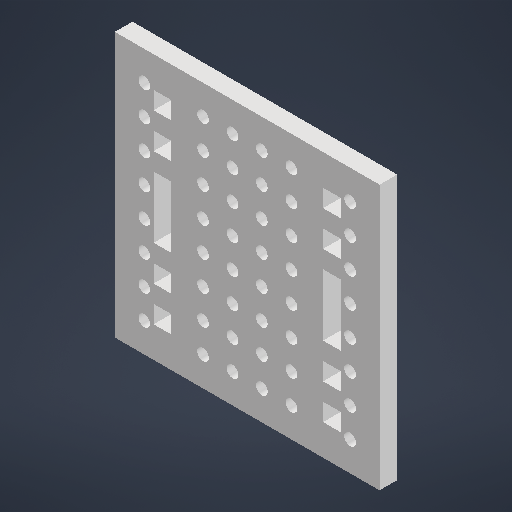
# Autodesk Inventor part: FootScrewplate
Saved by Autodesk Inventor 2027 (Build 310192000, 192)
## iProperties
Created: 2026-04-15
Part Number: FootScrewplate
Material: Generic
Document SubType Name: Modeling
Designer: Tueha
Density: 1 g/cm^3
Appearance: Default
Author: Tueha
Autodesk Inventor part; units mm, degrees
ref_plane "YZ Plane" through (0, 0, 0) normal (1, 0, 0) x (0, 1, 0)
ref_plane "XZ Plane" through (0, 0, 0) normal (0, 1, 0) x (-1, 0, 0)
ref_plane "XY Plane" through (0, 0, 0) normal (0, 0, 1) x (1, 0, 0)
sketch "Sketch1" plane through (0, 0, 0) normal (0, 0, 1) x (1, 0, 0)
  line L0 (-43.8671, 76.4402) -> (46.1329, 76.4402)
  line L1 (46.1329, 76.4402) -> (46.1329, -13.5598)
  line L2 (46.1329, -13.5598) -> (-43.8671, -13.5598)
  line L3 (-43.8671, -13.5598) -> (-43.8671, 76.4402)
  point P0 (0, 0)
  dimension "d0" = 90
  dimension "d1" = 90
  constraints: 8 end point, 2 parallel, 1 horizontal, 1 perpendicular
  measures "d0" distance of L1.end L2.end
  measures "d1" distance of L0.end L1.end
extrude "Extrusion1" add sketch "Sketch1" along normal blind 6
sketch "Sketch2" plane through (0, 0, 0) normal (0, 0, -1) x (-1, 0, 0)
  line L0 (24.6671, 8.9402) -> (30.6671, 8.9402) projected
  line L1 (30.6671, 8.9402) -> (30.6671, 2.9402) projected
  line L2 (30.6671, 2.9402) -> (24.6671, 2.9402) projected
  line L3 (24.6671, 8.9402) -> (24.6671, 2.9402) projected
  line L4 (30.6671, 14.9402) -> (24.6671, 14.9402) projected
  line L5 (24.6671, 20.9402) -> (24.6671, 14.9402) projected
  line L6 (30.6671, 20.9402) -> (24.6671, 20.9402) projected
  line L7 (30.6671, 20.9402) -> (30.6671, 14.9402) projected
  line L8 (24.6671, 47.9402) -> (30.6671, 47.9402) projected
  line L9 (30.6671, 41.9402) -> (30.6671, 47.9402) projected
  line L10 (24.6671, 41.9402) -> (30.6671, 41.9402) projected
  line L11 (24.6671, 41.9402) -> (24.6671, 47.9402) projected
  line L12 (24.6671, 59.9402) -> (30.6671, 59.9402) projected
  line L13 (30.6671, 53.9402) -> (30.6671, 59.9402) projected
  line L14 (30.6671, 53.9402) -> (24.6671, 53.9402) projected
  line L15 (24.6671, 53.9402) -> (24.6671, 59.9402) projected
  line L16 (-32.9329, 47.9402) -> (-26.9329, 47.9402) projected
  line L17 (-26.9329, 41.9402) -> (-26.9329, 47.9402) projected
  line L18 (-32.9329, 41.9402) -> (-26.9329, 41.9402) projected
  line L19 (-32.9329, 41.9402) -> (-32.9329, 47.9402) projected
  line L20 (-32.9329, 59.9402) -> (-26.9329, 59.9402) projected
  line L21 (-26.9329, 53.9402) -> (-26.9329, 59.9402) projected
  line L22 (-26.9329, 53.9402) -> (-32.9329, 53.9402) projected
  line L23 (-32.9329, 53.9402) -> (-32.9329, 59.9402) projected
  line L24 (-26.9329, 14.9402) -> (-32.9329, 14.9402) projected
  line L25 (-32.9329, 20.9402) -> (-32.9329, 14.9402) projected
  line L26 (-26.9329, 20.9402) -> (-32.9329, 20.9402) projected
  line L27 (-26.9329, 20.9402) -> (-26.9329, 14.9402) projected
  line L28 (-32.9329, 8.9402) -> (-26.9329, 8.9402) projected
  line L29 (-26.9329, 8.9402) -> (-26.9329, 2.9402) projected
  line L30 (-26.9329, 2.9402) -> (-32.9329, 2.9402) projected
  line L31 (-32.9329, 8.9402) -> (-32.9329, 2.9402) projected
  line L32 (-32.9329, 8.9402) -> (-26.9329, 8.9402)
  line L33 (-26.9329, 8.9402) -> (-26.9329, 14.9402)
  line L34 (-26.9329, 14.9402) -> (-32.9329, 14.9402)
  line L35 (-32.9329, 14.9402) -> (-32.9329, 8.9402)
  line L36 (-32.9329, 2.9402) -> (-26.9329, 2.9402)
  line L37 (-26.9329, 2.9402) -> (-26.9329, -3.0598)
  line L38 (-26.9329, -3.0598) -> (-32.9329, -3.0598)
  line L39 (-32.9329, -3.0598) -> (-32.9329, 2.9402)
  line L40 (-32.9329, 47.9402) -> (-26.9329, 47.9402)
  line L41 (-26.9329, 47.9402) -> (-26.9329, 53.9402)
  line L42 (-26.9329, 53.9402) -> (-32.9329, 53.9402)
  line L43 (-32.9329, 53.9402) -> (-32.9329, 47.9402)
  line L44 (-32.9329, 59.9402) -> (-26.9329, 59.9402)
  line L45 (-26.9329, 59.9402) -> (-26.9329, 65.9402)
  line L46 (-26.9329, 65.9402) -> (-32.9329, 65.9402)
  line L47 (-32.9329, 65.9402) -> (-32.9329, 59.9402)
  line L48 (24.6671, 47.9402) -> (30.6671, 47.9402)
  line L49 (30.6671, 47.9402) -> (30.6671, 53.9402)
  line L50 (30.6671, 53.9402) -> (24.6671, 53.9402)
  line L51 (24.6671, 53.9402) -> (24.6671, 47.9402)
  line L52 (24.6671, 59.9402) -> (30.6671, 59.9402)
  line L53 (30.6671, 59.9402) -> (30.6671, 65.9402)
  line L54 (30.6671, 65.9402) -> (24.6671, 65.9402)
  line L55 (24.6671, 65.9402) -> (24.6671, 59.9402)
  line L56 (24.6671, 8.9402) -> (30.6671, 8.9402)
  line L57 (30.6671, 8.9402) -> (30.6671, 14.9402)
  line L58 (30.6671, 14.9402) -> (24.6671, 14.9402)
  line L59 (24.6671, 14.9402) -> (24.6671, 8.9402)
  line L60 (24.6671, 2.9402) -> (30.6671, 2.9402)
  line L61 (30.6671, 2.9402) -> (30.6671, -3.0598)
  line L62 (30.6671, -3.0598) -> (24.6671, -3.0598)
  line L63 (24.6671, -3.0598) -> (24.6671, 2.9402)
  point P0 (0, 0)
  dimension "d4" = 6
  dimension "d5" = 6
  dimension "d6" = 6
  dimension "d7" = 6
  dimension "d8" = 6
  dimension "d9" = 6
  dimension "d10" = 6
  dimension "d11" = 6
  dimension "d12" = 6
  dimension "d13" = 6
  constraints: 64 end point, 16 parallel, 8 horizontal, 8 perpendicular
  measures "d4" distance of L37.end L38.end
  measures "d5" distance of L36.end L37.end
  measures "d6" distance of L46.end L45.end
  measures "d7" distance of L45.end L44.end
  measures "d8" distance of L54.end L53.end
  measures "d9" distance of L53.end L52.end
  measures "d10" distance of L58.end L4.start
  measures "d11" distance of L4.start L56.end
  measures "d12" distance of L61.end L62.end
  measures "d13" distance of L60.end L61.end
extrude "Extrusion2" cut sketch "Sketch2" against normal blind 6 contours L59 L4 L57 L0 | L2 L61 L62 L63 | L51 L14 L49 L8 | L55 L54 L53 L12 | L43 L22 L41 L16 | L47 L46 L45 L20 | L33 L28 L35 L24 | L37 L38 L39 L30
sketch "Sketch3" plane through (0, 0, 6) normal (0, 0, 1) x (1, 0, 0)
  circle A0 centre (-33.8671, -3.5598) radius 2
  line L0 (-43.8671, 76.4402) -> (-43.8671, -13.5598) projected
  line L1 (-43.8671, -13.5598) -> (46.1329, -13.5598) projected
  circle A1 centre (-33.8671, 6.4402) radius 2
  circle A2 centre (-33.8671, 16.4402) radius 2
  circle A3 centre (-33.8671, 26.4402) radius 2
  circle A4 centre (-33.8671, 36.4402) radius 2
  circle A5 centre (-33.8671, 46.4402) radius 2
  circle A6 centre (-33.8671, 56.4402) radius 2
  circle A7 centre (-33.8671, 66.4402) radius 2
  circle A8 centre (-23.8671, -3.5598) radius 2
  circle A9 centre (-23.8671, 6.4402) radius 2
  circle A10 centre (-23.8671, 16.4402) radius 2
  circle A11 centre (-23.8671, 26.4402) radius 2
  circle A12 centre (-23.8671, 36.4402) radius 2
  circle A13 centre (-23.8671, 46.4402) radius 2
  circle A14 centre (-23.8671, 56.4402) radius 2
  circle A15 centre (-23.8671, 66.4402) radius 2
  circle A16 centre (-13.8671, -3.5598) radius 2
  circle A17 centre (-13.8671, 6.4402) radius 2
  circle A18 centre (-13.8671, 16.4402) radius 2
  circle A19 centre (-13.8671, 26.4402) radius 2
  circle A20 centre (-13.8671, 36.4402) radius 2
  circle A21 centre (-13.8671, 46.4402) radius 2
  circle A22 centre (-13.8671, 56.4402) radius 2
  circle A23 centre (-13.8671, 66.4402) radius 2
  circle A24 centre (-3.8671, -3.5598) radius 2
  circle A25 centre (-3.8671, 6.4402) radius 2
  circle A26 centre (-3.8671, 16.4402) radius 2
  circle A27 centre (-3.8671, 26.4402) radius 2
  circle A28 centre (-3.8671, 36.4402) radius 2
  circle A29 centre (-3.8671, 46.4402) radius 2
  circle A30 centre (-3.8671, 56.4402) radius 2
  circle A31 centre (-3.8671, 66.4402) radius 2
  circle A32 centre (6.1329, -3.5598) radius 2
  circle A33 centre (6.1329, 6.4402) radius 2
  circle A34 centre (6.1329, 16.4402) radius 2
  circle A35 centre (6.1329, 26.4402) radius 2
  circle A36 centre (6.1329, 36.4402) radius 2
  circle A37 centre (6.1329, 46.4402) radius 2
  circle A38 centre (6.1329, 56.4402) radius 2
  circle A39 centre (6.1329, 66.4402) radius 2
  circle A40 centre (16.1329, -3.5598) radius 2
  circle A41 centre (16.1329, 6.4402) radius 2
  circle A42 centre (16.1329, 16.4402) radius 2
  circle A43 centre (16.1329, 26.4402) radius 2
  circle A44 centre (16.1329, 36.4402) radius 2
  circle A45 centre (16.1329, 46.4402) radius 2
  circle A46 centre (16.1329, 56.4402) radius 2
  circle A47 centre (16.1329, 66.4402) radius 2
  circle A48 centre (26.1329, -3.5598) radius 2
  circle A49 centre (26.1329, 6.4402) radius 2
  circle A50 centre (26.1329, 16.4402) radius 2
  circle A51 centre (26.1329, 26.4402) radius 2
  circle A52 centre (26.1329, 36.4402) radius 2
  circle A53 centre (26.1329, 46.4402) radius 2
  circle A54 centre (26.1329, 56.4402) radius 2
  circle A55 centre (26.1329, 66.4402) radius 2
  circle A56 centre (36.1329, -3.5598) radius 2
  circle A57 centre (36.1329, 6.4402) radius 2
  circle A58 centre (36.1329, 16.4402) radius 2
  circle A59 centre (36.1329, 26.4402) radius 2
  circle A60 centre (36.1329, 36.4402) radius 2
  circle A61 centre (36.1329, 46.4402) radius 2
  circle A62 centre (36.1329, 56.4402) radius 2
  circle A63 centre (36.1329, 66.4402) radius 2
  point P0 (0, 0)
  dimension "d16" = 4
  dimension "d18" = 10
  dimension "d21" = 10
  dimension "d24" = 10
  dimension "d27" = 10
  constraints: 64 centre point, 1 horizontal, 1 vertical, 126 other
  measures "d16" diameter of A0
  measures "d18" distance from line of L1 A0.centre
  measures "d21" distance of A0.centre A1.centre
  measures "d24" distance of A0.centre A8.centre
  measures "d27" distance from line of L0 A0.centre
extrude "Extrusion3" cut sketch "Sketch3" against normal blind 6 contours A0 | A1 | A2 | A3 | A4 | A5 | A6 | A7 | A16 | A17 | A18 | A19 | A20 | A21 | A22 | A23 | A24 | A25 | A26 | A27 | A28 | A29 | A30 | A31 | A32 | A33 | A34 | A35 | A36 | A37 | A38 | A39 | A40 | A41 | A42 | A43 | A44 | A45 | A46 | A47 | A56 | A57 | A58 | A59 | A60 | A61 | A62 | A63
sketch "Sketch4" plane through (0, 0, 0) normal (0, 0, -1) x (-1, 0, 0)
  line L0 (-32.9329, 20.9402) -> (-32.9329, 41.9402) projected
  line L1 (-32.9329, 20.9402) -> (-32.9329, 41.9402) projected
  line L2 (-32.9329, 41.9402) -> (-26.9329, 41.9402) projected
  line L3 (-32.9329, 41.9402) -> (-26.9329, 41.9402) projected
  line L4 (-32.9329, 41.9402) -> (-26.9329, 41.9402) projected
  line L5 (-32.9329, 20.9402) -> (-32.9329, 41.9402) projected
  line L6 (-26.9329, 41.9402) -> (-26.9329, 20.9402) projected
  line L7 (-26.9329, 20.9402) -> (-32.9329, 20.9402) projected
  point P0 (0, 0)
extrude "Extrusion4" cut sketch "Sketch4" against normal blind 6
sketch "Sketch5" plane through (0, 0, 6) normal (0, 0, 1) x (1, 0, 0)
  line L0 (-30.6671, 41.9402) -> (-30.6671, 20.9402) projected
  line L1 (-30.6671, 20.9402) -> (-24.6671, 20.9402) projected
  line L2 (-24.6671, 20.9402) -> (-24.6671, 41.9402) projected
  line L3 (-24.6671, 41.9402) -> (-30.6671, 41.9402) projected
  point P0 (0, 0)
extrude "Extrusion5" cut sketch "Sketch5" against normal blind 6
body "Solid1"
